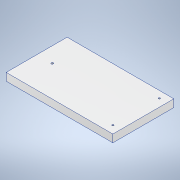
# Autodesk Inventor part: Carrier Plate V1
Saved by Autodesk Inventor 2022 (Build 260153000, 153)
## iProperties
Created: 2022-04-14
Part Number: Carrier Plate V1
Material: Aluminum 6061
Document SubType Name: Modeling
Designer: Caleb
Density: 2.7 g/cm^3
Appearance: Aluminum - Flat
Author: Caleb
Autodesk Inventor part; units mm, degrees
ref_plane "YZ Plane" through (0, 0, 0) normal (1, 0, 0) x (0, 1, 0)
ref_plane "XZ Plane" through (0, 0, 0) normal (0, 1, 0) x (-1, 0, 0)
ref_plane "XY Plane" through (0, 0, 0) normal (0, 0, 1) x (1, 0, 0)
sketch "Sketch1" plane through (0, 0, 0) normal (0, 1, 0) x (-1, 0, 0)
  line L0 (-44.45, -25.4) -> (44.45, -25.4)
  line L1 (44.45, -25.4) -> (44.45, 25.4)
  line L2 (44.45, 25.4) -> (-44.45, 25.4)
  line L3 (-44.45, 25.4) -> (-44.45, -25.4)
  line L4 (-44.45, -25.4) -> (44.45, 25.4) construction
  line L5 (44.45, -25.4) -> (-44.45, 25.4) construction
  point P0 (0, 0)
  dimension "d0" = 88.9
  dimension "d1" = 50.8
  constraints: 12 end point, 2 midpoint, 2 parallel, 1 horizontal, 1 perpendicular
  measures "d0" distance of L2.end L1.end
  measures "d1" distance of L1.end L0.end
extrude "Extrusion1" add sketch "Sketch1" along normal blind 6.35
sketch "Sketch2" plane through (0, 6.35, 0) normal (0, 1, 0) x (1, 0, 0)
  line L0 (44.45, -25.4) -> (44.45, 25.4) projected
  line L1 (-44.45, -25.4) -> (44.45, -25.4) projected
  point P0 (0, 0)
  point P1 (38.1, -19.05)
  point P2 (38.1, 19.685)
  dimension "d4" = 6.35
  dimension "d5" = 38.735
  dimension "d6" = 6.35
  constraints: 1 vertical alignment
  measures "d4" distance from line of L0 point (38.1, -19.05)
  measures "d5" distance of point (38.1, -19.05) point (38.1, 19.685)
  measures "d6" distance from line of L1 point (38.1, -19.05)
hole "Hole1" at (38.1, 6.35, 19.05) at (38.1, 6.35, -19.685) direction (0, -1, 0) diameter 1.4249 end through all thread size "1-64 UNC" class "2B" standard "ANSI Unified Screw Threads"
sketch "Sketch3" plane through (0, 6.35, 0) normal (0, 1, 0) x (1, 0, 0)
  line L0 (-44.45, 25.4) -> (-44.45, -25.4) projected
  circle A0 centre (38.1, 19.685) radius 0.7125 projected
  circle A1 centre (38.1, -19.05) radius 0.7125 projected
  line L1 (-44.45, -25.4) -> (44.45, -25.4) projected
  point P0 (0, 0)
  point P1 (-31.75, 0.3175)
  dimension "d14" = 12.7
  dimension "d15" = 25.7175
  measures "d14" distance from line of L0 point (-31.75, 0.318)
  measures "d15" distance from line of L1 point (-31.75, 0.318)
hole "Hole2" at (-31.75, 6.35, -0.3175) direction (0, -1, 0) diameter 1.6942 end through all thread size "2-56 UNC" class "2B" standard "ANSI Unified Screw Threads"
body "Solid1"
